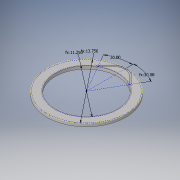
# Autodesk Inventor part: NewCam02
Saved by Autodesk Inventor 2016 (Build 200138000, 138)
## iProperties
Created: 2015-07-23
Part Number: NewCam02
Material: Generic
Document SubType Name: Modeling
Designer: steele
Density: 1 g/cm^3
Appearance: Default
Author: steele
Autodesk Inventor part; units mm, degrees
sketch "Sketch1" plane through (0, 0, 0) normal (0, 1, 0) x (-1, 0, 0)
  circle A0 centre (0, 0) radius 139.7
  circle A1 centre (0, 0) radius 177.8
  dimension "innerDiameter" = 279.4
  dimension "outerDiameter" = 355.6
  constraints: 2 centre point, 2 coincident
  measures "innerDiameter" diameter of A0
  measures "outerDiameter" diameter of A1
extrude "Extrusion1" add sketch "Sketch1" against normal blind 12.7
sketch "Sketch5" plane through (0, 0, 0) normal (0, 1, 0) x (1, 0, 0)
  line L0 (0, 0) -> (-88.9, 153.9793) construction
  circle A0 centre (0, 0) radius 177.8 construction
  line L1 (0, 0) -> (88.9, 153.9793) construction
  line L2 (0, 0) -> (0, 177.8) construction
  circle A1 centre (0, 0) radius 142.875 construction
  circle A2 centre (0, 0) radius 174.625 construction
  point P0 (71.4375, 123.7334)
  point P1 (0, 174.625)
  point P2 (-71.4375, 123.7334)
  dimension "camOuterDiameter" = 349.25
  dimension "arcForCam" = 30
  dimension "d12" = 30
  dimension "camInnerDiameter" = 285.75
  constraints: 6 end point, 5 point on circle, 3 point on line, 2 coincident, 1 centre point, 1 vertical, 1 vertical alignment, 2 other
  measures "arcForCam" angle of L0 L2
  measures "d12" angle of L1 L2
  measures "camInnerDiameter" diameter of A1
ref_plane "Work Plane3" through (0, 0, 0) normal (0.8660254, 0, 0.5) x (0.5, 0, -0.8660254)
ref_plane "Work Plane4" through (0, 0, 0) normal (-1, 0, 0) x (0, 0, -1)
ref_plane "Work Plane5" through (0, 0, 0) normal (0.8660254, 0, -0.5) x (-0.5, 0, -0.8660254)
sketch "Sketch10" plane through (0, 0, 0) normal (0.8660254, 0, 0.5) x (0.5, 0, -0.8660254)
  line L0 (-177.8, 0) -> (177.8, 0) projected
  circle A0 centre (142.875, 0) radius 3.175
  point P0 (0, 0)
  dimension "camDiameter" = 6.35
  dimension "d30" = 142.875
  constraints: 1 centre point, 1 point on line
  measures "camDiameter" diameter of A0
  measures "d30" distance of A0.centre point (0, 0)
sketch "Sketch12" plane through (0, 0, 0) normal (-1, 0, 0) x (0, 0, -1)
  circle A0 centre (174.625, 0) radius 3.175
  point P0 (0, 0)
  dimension "d31" = 174.625
  dimension "d32" = 6.35
  constraints: 1 centre point
  measures "d31" distance of A0.centre point (0, 0)
  measures "d32" diameter of A0
sketch "Sketch13" plane through (0, 0, 0) normal (0.8660254, 0, -0.5) x (-0.5, 0, -0.8660254)
  circle A0 centre (142.875, 0) radius 3.175
  point P0 (0, 0)
  dimension "d33" = 6.35
  dimension "d34" = 142.875
  constraints: 1 centre point
  measures "d33" diameter of A0
  measures "d34" distance of A0.centre point (0, 0)
loft "Loft2" cut profiles "Sketch10", "Sketch12", "Sketch13"
equation "\"d12\" = arcForCam"
equation "\"d30\" = 0.5 * camInnerDiameter"
equation "\"d31\" = 0.5 * camOuterDiameter"
equation "\"d32\" = camDiameter"
equation "\"d33\" = camDiameter"
equation "\"d34\" = 0.5 * camInnerDiameter"
body "Solid1"
